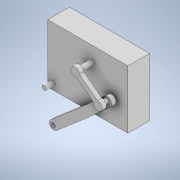
# Autodesk Inventor part: Деталь3
Saved by Autodesk Inventor 2020.1 (Build 241239000, 239)
## iProperties
Created: 2021-11-17
Part Number: Деталь3
Material: Типовые
Document SubType Name: Modeling
Designer: Ni3na
Density: 1 g/cm^3
Appearance: По умолчанию
Author: Ni3na
Autodesk Inventor part; units mm, degrees
ref_plane "YZ Plane" through (0, 0, 0) normal (1, 0, 0) x (0, 1, 0)
ref_plane "XZ Plane" through (0, 0, 0) normal (0, 1, 0) x (-1, 0, 0)
ref_plane "XY Plane" through (0, 0, 0) normal (0, 0, 1) x (1, 0, 0)
sketch "Эскиз1" plane through (0, 0, 0) normal (0, 0, 1) x (1, 0, 0)
  line L0 (10.0582, -8.8009) -> (-16.8718, -8.8009)
  line L1 (-16.8718, -8.8009) -> (-16.8718, 8.0709)
  line L2 (-16.8718, 8.0709) -> (10.0582, 8.0709)
  line L3 (10.0582, 8.0709) -> (10.0582, -8.8009)
  point P0 (0, 0)
  constraints: 8 end point, 2 parallel, 1 horizontal, 1 perpendicular
extrude "Выдавливание1" add sketch "Эскиз1" along normal blind 10
sketch "Эскиз2" plane through (0, 0, 10) normal (0, 0, 1) x (1, 0, 0)
  circle A0 centre (4.6641, -5.9619) radius 1
  circle A1 centre (-14.4383, -5.9619) radius 1
  point P0 (0, 0)
  dimension "d2" = 2
  dimension "d3" = 2
  constraints: 2 centre point
  measures "d2" diameter of A0
  measures "d3" diameter of A1
extrude "Выдавливание2" add sketch "Эскиз2" along normal blind 2
sketch "Эскиз3" plane through (4.6641, -5.9619, 12) normal (0, 0, 1) x (1, 0, 0)
  circle A0 centre (0, 0) radius 1 projected
  circle A1 centre (0, 0) radius 2
  circle A2 centre (-14.7836, -12.664) radius 2
  line L0 (-1.2061, 1.5954) -> (-15.8126, -10.949)
  line L1 (-13.5836, -14.264) -> (1.0265, -1.7165)
  point P0 (-4.6641, 5.9619)
  dimension "d6" = 4
  dimension "d7" = 4
  constraints: 4 end point, 4 point on circle, 2 centre point, 1 coincident, 1 parallel
  measures "d6" diameter of A1
  measures "d7" diameter of A2
extrude "Выдавливание3" add sketch "Эскиз3" along normal blind 2
sketch "Эскиз4" plane through (-14.4383, -5.9619, 12) normal (0, 0, 1) x (1, 0, 0)
  circle A0 centre (0, 0) radius 1
  point P0 (14.4383, 5.9619)
  constraints: 1 centre point
extrude "Выдавливание4" add sketch "Эскиз4" along normal blind 4
sketch "Эскиз5" plane through (4.6641, -5.9619, 14) normal (0, 0, 1) x (1, 0, 0)
  circle A0 centre (-10.7969, -8.6603) radius 1
  point P0 (-4.6641, 5.9619)
  dimension "d12" = 2
  constraints: 1 centre point
  measures "d12" diameter of A0
extrude "Выдавливание5" add sketch "Эскиз5" along normal blind 2
sketch "Эскиз6" plane through (4.6641, -5.9619, 14) normal (0, 0, 1) x (1, 0, 0)
  circle A0 centre (-15.0265, -12.7992) radius 1
  point P0 (-4.6641, 5.9619)
  dimension "d15" = 2
  constraints: 1 centre point
  measures "d15" diameter of A0
extrude "Выдавливание6" cut sketch "Эскиз6" against normal blind 10
sketch "Эскиз7" plane through (-14.4383, -5.9619, 16) normal (0, 0, 1) x (1, 0, 0)
  circle A0 centre (0, 0) radius 2
  circle A1 centre (8.3055, -8.6603) radius 1 projected
  circle A2 centre (8.3055, -8.6603) radius 2
  line L0 (7.3055, -6.9282) -> (1.7093, -1.0384)
  line L1 (6.6268, -7.5731) -> (1.0492, -1.7027)
  point P0 (14.4383, 5.9619)
  dimension "d18" = 4
  dimension "d19" = 4
  constraints: 4 end point, 4 point on circle, 2 centre point, 1 coincident, 1 parallel
  measures "d18" diameter of A0
  measures "d19" diameter of A2
extrude "Выдавливание7" add sketch "Эскиз7" along normal blind 2 contours A0 | A0 L0 A2 L1 | A2 | A1
sketch "Эскиз8" plane through (-14.4383, -5.9619, 18) normal (0, 0, 1) x (1, 0, 0)
  circle A0 centre (0, 0) radius 1
  point P0 (14.4383, 5.9619)
  constraints: 1 centre point
extrude "Выдавливание8" cut sketch "Эскиз8" against normal blind 1
chamfer "Фаска1" distance 0.3 angle 45 4 edges at (-9.9309, -9.9452, 18) (-9.9309, -9.9452, 16) (-10.6004, -10.5998, 16) (-10.6004, -10.5998, 18)
sketch "Эскиз9" plane through (-14.4383, -5.9619, 18) normal (0, 0, 1) x (1, 0, 0)
  line L0 (-16.7765, 10.1097) -> (30.4978, 10.1097)
  line L1 (30.4978, 10.1097) -> (30.4978, -12.7564)
  line L2 (30.4978, -12.7564) -> (-16.7765, -12.7564)
  line L3 (-16.7765, -12.7564) -> (-16.7765, 10.1097)
  point P0 (14.4383, 5.9619)
  constraints: 8 end point, 2 parallel, 1 horizontal, 1 perpendicular
extrude "Выдавливание9" cut sketch "Эскиз9" against normal blind 4
sketch "Эскиз10" plane through (10.0582, -8.8009, 0) normal (1, 0, 0) x (0, 0, -1)
  line L0 (0, 0) -> (0, 16.8718) projected
  line L1 (-10, 0) -> (-10, 16.8718) projected
  line L2 (0, 0) -> (-10, 0)
  line L3 (-10, 0) -> (-10, 16.8718)
  line L4 (-10, 16.8718) -> (0, 16.8718)
  line L5 (0, 16.8718) -> (0, 0)
  point P0 (0, 8.8009)
  constraints: 8 end point, 2 parallel, 1 horizontal, 1 perpendicular
extrude "Выдавливание10" add sketch "Эскиз10" along normal blind 10
sketch "Эскиз11" plane through (4.6641, -5.9619, 14) normal (0, 0, 1) x (1, 0, 0)
  circle A0 centre (9.9064, 8.993) radius 2
  arc A1 (1.0265, -1.7165) -> (-1.2061, 1.5954) centre (0, 0) ccw projected
  line L0 (8.4408, 10.3539) -> (-1.2061, 1.5954)
  line L1 (-1.2061, 1.5954) -> (1.0265, -1.7165)
  line L2 (1.0265, -1.7165) -> (11.2465, 7.5083)
  point P0 (-4.6641, 5.9619)
  point P1 (1.6027, -1.1964)
  dimension "d31" = 4
  constraints: 6 end point, 2 point on circle, 1 centre point, 1 tangent
  measures "d31" diameter of A0
extrude "Выдавливание11" add sketch "Эскиз11" against normal blind 2 contours A0 | A0 L2 A1 L0
sketch "Эскиз12" plane through (-16.8718, 8.0709, 10) normal (0, 1, 0) x (1, 0, 0)
  line L0 (0, 10) -> (36.9299, 10) projected
  line L1 (0, 0) -> (36.9299, 0) projected
  line L2 (0, 10) -> (36.9299, 10)
  line L3 (36.9299, 10) -> (36.9299, 0)
  line L4 (36.9299, 0) -> (0, 0)
  line L5 (0, 0) -> (0, 10)
  point P0 (16.8718, 10)
  constraints: 8 end point, 2 parallel, 1 horizontal, 1 perpendicular
extrude "Выдавливание12" add sketch "Эскиз12" along normal blind 10
sketch "Эскиз13" plane through (0, 0, 10) normal (0, 0, 1) x (1, 0, 0)
  circle A0 centre (3.7224, 11.5394) radius 1
  point P0 (0, 0)
  dimension "d36" = 2
  constraints: 1 centre point
  measures "d36" diameter of A0
extrude "Выдавливание13" add sketch "Эскиз13" along normal blind 6
sketch "Эскиз14" plane through (4.6641, -5.9619, 14) normal (0, 0, 1) x (1, 0, 0)
  circle A0 centre (9.5274, 9.2057) radius 1
  point P0 (-4.6641, 5.9619)
  dimension "d39" = 2
  constraints: 1 centre point
  measures "d39" diameter of A0
extrude "Выдавливание14" add sketch "Эскиз14" along normal blind 2
sketch "Эскиз15" plane through (3.7224, 11.5394, 16) normal (0, 0, 1) x (1, 0, 0)
  circle A0 centre (0, 0) radius 1 projected
  circle A1 centre (0, 0) radius 2
  circle A2 centre (10.469, -8.2956) radius 1 projected
  circle A3 centre (10.469, -8.2956) radius 2
  line L0 (10.314, -6.3017) -> (2, 0)
  line L1 (9.3825, -7.1474) -> (-0.2644, -15.9059) projected
  line L2 (8.4993, -7.9493) -> (0.5405, -1.9256)
  point P0 (-3.7224, -11.5394)
  dimension "d42" = 4
  dimension "d43" = 4
  constraints: 4 end point, 4 point on circle, 2 centre point, 2 coincident, 1 point on line
  measures "d42" diameter of A1
  measures "d43" diameter of A3
extrude "Выдавливание15" add sketch "Эскиз15" along normal blind 2 contours A0 | A1 | L0 A3 L2 A1 | A3 | A2
